outside encoder right (Autodesk Fusion 360 design; units mm, degrees)
Autodesk Fusion 360 part; units mm, degrees
note: some values were not read from the file. Set by a fixed rule: which sketch regions a step uses.
sketch "Sketch1" plane through (0, -20.5, 31.25) normal (0, 0, 1) x (-1, 0, 0)
  circle A0 centre (0, -20.5) radius 3.95
  circle A1 centre (0, -20.5) radius 4.05
  circle A2 centre (0, -20.5) radius 6
  line L0 (12.5, 14.5) -> (-12.5, 14.5)
  line L1 (12.5, 14.5) -> (12.5, -26.5)
  line L2 (12.5, -26.5) -> (-12.5, -26.5)
  line L3 (-12.5, -26.5) -> (-12.5, 14.5)
  circle A3 centre (-8.2191, 7.965) radius 1.725
  circle A4 centre (7.8309, -8.085) radius 1.725
  circle A5 centre (-8.1691, -8.085) radius 1.725
  circle A6 centre (7.8309, 7.965) radius 1.725
  arc A7 (-11.6441, -8.0959) -> (-8.1691, -11.56) centre (-8.1691, -8.085) ccw
  line L4 (-8.1691, -11.56) -> (7.8309, -11.56)
  arc A8 (7.8309, -11.56) -> (11.3059, -8.085) centre (7.8309, -8.085) ccw
  line L5 (11.3059, -8.085) -> (11.3059, 7.965)
  arc A9 (11.3059, 7.965) -> (7.8309, 11.44) centre (7.8309, 7.965) ccw
  line L6 (7.8309, 11.44) -> (-8.2191, 11.44)
  arc A10 (-8.2191, 11.44) -> (-11.6941, 7.9541) centre (-8.2191, 7.965) ccw
  line L7 (-11.6941, 7.9541) -> (-11.6441, -8.0959)
  line L8 (11.4059, -8.085) -> (11.4059, 7.965)
  arc A11 (11.4059, 7.965) -> (7.8309, 11.54) centre (7.8309, 7.965) ccw
  line L9 (7.8309, 11.54) -> (-8.2191, 11.54)
  arc A12 (-8.2191, 11.54) -> (-11.7941, 7.9538) centre (-8.2191, 7.965) ccw
  line L10 (-11.7941, 7.9538) -> (-11.7441, -8.0962)
  arc A13 (-11.7441, -8.0962) -> (-8.1691, -11.66) centre (-8.1691, -8.085) ccw
  line L11 (-8.1691, -11.66) -> (7.8309, -11.66)
  arc A14 (7.8309, -11.66) -> (11.4059, -8.085) centre (7.8309, -8.085) ccw
  dimension "d108" = 8.1
  dimension "d109" = 12
  dimension "d110" = 0.1
  constraint concentric A0 A1
  constraint concentric A1 A2
  constraint coincident L0.start L1.start
  constraint perpendicular L0 L1
  constraint perpendicular L1 L2
  constraint coincident L0.end L3.end
  constraint tangent A2 L2
  constraint perpendicular L2 L3
  measures "d108" diameter of A1
  measures "d109" diameter of A2
extrude "Extrude1" add sketch "Sketch1" along normal blind 3.5 and the other way blind 2.5 contours A2 | L0 L1 L2 L3
extrude "Extrude2" add sketch "Sketch1" against normal blind 3.5 contours A2
sketch "Sketch2" plane through (0, 6, 0) normal (0, 1, 0) x (-1, 0, 0)
  line L0 (12.5, 28.75) -> (12.5, 34.75)
  line L1 (12.5, 34.75) -> (-12.5, 34.75)
  line L2 (-12.5, 34.75) -> (-12.5, 28.75)
  line L3 (-12.5, 28.75) -> (0, 28.75)
  line L4 (0, 28.75) -> (12.5, 28.75)
  circle A0 centre (-25, 13.25) radius 3
  line L5 (0, 34.75) -> (0, 28.75)
  line L6 (-12.5, 28.75) -> (-20, 28.75)
  circle A1 centre (-25, 13.25) radius 5
  line L7 (-20, 28.75) -> (-20, 13.25)
  line L8 (-12.5, 34.75) -> (-26, 34.75)
  line L9 (-26, 34.75) -> (-26, 13.25)
  line L10 (-28.5355, 16.7855) -> (-26, 19.3211)
  line L11 (12.5, 34.75) -> (26, 34.75)
  line L12 (12.5, 28.75) -> (20, 28.75)
  line L13 (20, 28.75) -> (20, 13.25)
  line L14 (26, 34.75) -> (26, 13.25)
  line L15 (28.5355, 16.7855) -> (26, 19.3211)
  circle A2 centre (25, 13.25) radius 5
  circle A3 centre (25, 13.25) radius 3
  point P0 (12.5, 34.75)
  dimension "d117" = 2
  dimension "d118" = 6
  dimension "d119" = 45
  constraint midpoint L1 L5.start
  constraint coincident L3.end L4.start
  constraint coincident L2.end L3.start
  constraint perpendicular L2 L6
  constraint coincident A1 L7.end
  constraint tangent A1 L7
  constraint perpendicular L6 L7
  constraint coincident A1 L10.start
  constraint coincident L9 L10.end
  constraint tangent A1 L10
  constraint symmetric A0 L5 A3
  constraint symmetric L5 L2.end L0.start
  constraint symmetric L5 L6.end L12.end
  constraint symmetric L5 A1 A2
  constraint symmetric L5 L7.end L13.end
  constraint symmetric L5 L1.end P0
  constraint symmetric L5 L8.end L11.end
  constraint symmetric L5 L9.end L14.end
  constraint symmetric L5 L10.start L15.start
  constraint symmetric L5 L10.end L15.end
  constraint coincident P0 L0.end
  measures "d119" angle of L9 L10
extrude "Extrude3" add sketch "Sketch2" along normal blind 10 from surface at -21 contours L0 L11 L12 L13 L14 A2 | L2 L6 A1 L7 L8 L9 | A2 | L14 L15 A2 | A1 | A1 L9 L10
extrude "Extrude4" cut 2 faces at (24, -15, 27.607) (-24, -15, 27.607) along direction (0, 1, 0) blind 0.1
extrude "Extrude5" cut 1 faces at (24, -14.9, 27.607) along direction (0, 1, 0) blind 10
